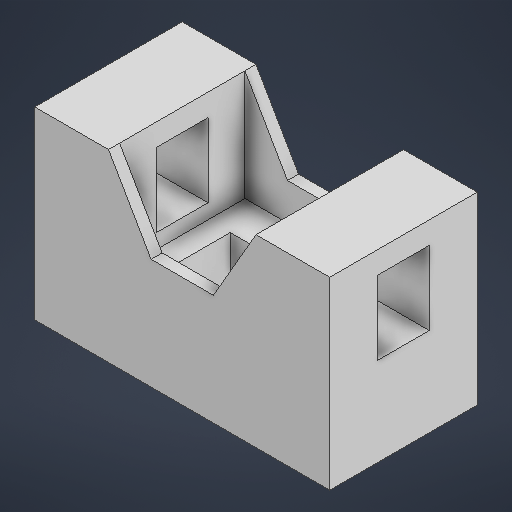
# Autodesk Inventor part: uhelnik_30x30_M6
Saved by Autodesk Inventor 2025.1 (Build 291241000, 241)
## iProperties
Created: 2024-12-28
Part Number: uhelnik_30x30_M6
Material: Všeobecné
Document SubType Name: Modeling
Designer: lukas
Density: 1 g/cm^3
Appearance: Výchozí
Author: lukas
## iProperties of the stored document uhelnik_30x30_3D tisk.ipt
Created: 2024-12-28
Part Number: uhelnik_30x30_3D tisk
Material: Všeobecné
Document SubType Name: Modeling
Designer: lukas
Density: 1 g/cm^3
Appearance: Výchozí
Author: lukas
Autodesk Inventor part; units mm, degrees
ref_plane "YZ Plane" through (0, 0, 0) normal (1, 0, 0) x (0, 1, 0)
ref_plane "XZ Plane" through (0, 0, 0) normal (0, 1, 0) x (-1, 0, 0)
ref_plane "XY Plane" through (0, 0, 0) normal (0, 0, 1) x (1, 0, 0)
sketch "Náčrt1" plane through (0, 0, 0) normal (0, 0, 1) x (1, 0, 0)
  line L0 (0, 17.5) -> (0, -17.5) projected
  line L1 (-28, 0) -> (28, 0) projected
  line L2 (-20, 12.5) -> (20, 12.5)
  line L3 (20, 12.5) -> (20, -12.5)
  line L4 (20, -12.5) -> (-20, -12.5)
  line L5 (-20, -12.5) -> (-20, 12.5)
  point P0 (0, 0)
  dimension "d0" = 40
  dimension "d1" = 25
  constraints: 8 end point, 2 parallel, 1 horizontal, 1 perpendicular, 2 other
  measures "d0" distance of L3.end L4.end
  measures "d1" distance of L2.end L3.end
extrude "Vysunutí1" add sketch "Náčrt1" along normal mid plane 20
sketch "Náčrt2" plane through (-20, 12.5, -10) normal (0, 1, 0) x (1, 0, 0)
  line L0 (0, 0) -> (40, 0) projected
  line L1 (0, 0) -> (0, -20) projected
  line L2 (40, -20) -> (0, -20) projected
  line L3 (40, 0) -> (40, -20) projected
  line L4 (-8, -10) -> (48, -10) projected
  line L5 (20, 4) -> (20, -24) projected
  line L6 (10, -18.5) -> (30, -18.5)
  line L7 (30, -18.5) -> (30, -1.5)
  line L8 (30, -1.5) -> (10, -1.5)
  line L9 (10, -1.5) -> (10, -18.5)
  point P0 (20, -10)
  dimension "d4" = 17
  dimension "d5" = 20
  constraints: 8 end point, 3 parallel, 1 horizontal, 1 perpendicular, 2 other
  measures "d4" distance of L8.end L6.start
  measures "d5" distance between parallel lines of L7 L9
extrude "Vysunutí2" cut sketch "Náčrt2" against normal blind 15 contours L8 L7 L4 L5 | L5 L4 L9 L8 | L4 L5 L6 L9 | L4 L7 L6 L5
sketch "Náčrt3" plane through (0, 0, 10) normal (0, 0, 1) x (1, 0, 0)
  line L0 (-20, -12.5) -> (20, -12.5) projected
  line L1 (20, -12.5) -> (20, 12.5) projected
  line L2 (20, 12.5) -> (-20, 12.5) projected
  line L3 (-20, 12.5) -> (-20, -12.5) projected
  line L4 (-10, 12.5) -> (-10, -2.5) projected
  line L5 (10, 12.5) -> (10, -2.5) projected
  line L6 (10, -2.5) -> (-10, -2.5) projected
  line L7 (-28, 0) -> (28, 0) projected
  line L8 (0, -17.5) -> (0, 17.5) projected
  line L9 (-10, 12.5) -> (-4.2265, 2.5)
  line L10 (-4.2265, 2.5) -> (4.2265, 2.5)
  line L11 (-20, 12.5) -> (20, 12.5) projected
  line L12 (4.2265, 2.5) -> (10, 12.5)
  line L13 (-10, 12.5) -> (10, 12.5)
  point P0 (0, 0)
  point P1 (0, 3.8397)
  dimension "d8" = 5
  dimension "d9" = 30
  dimension "d10" = 30
  constraints: 8 end point, 1 collinear, 1 parallel
  measures "d8" distance between parallel lines of L6 L10
  measures "d9" angle of L5 L12
  measures "d10" angle of L4 L9
extrude "Vysunutí3" cut sketch "Náčrt3" against normal through all contours L2 L8 L10 L9 | L8 L2 L12 L10
sketch "Náčrt5" plane through (20, -12.5, 10) normal (1, 0, 0) x (0, 0, -1)
  line L0 (20, 25) -> (0, 25) projected
  line L1 (0, 0) -> (0, 25) projected
  line L2 (20, 0) -> (0, 0) projected
  line L3 (20, 25) -> (20, 0) projected
  line L4 (18.5, 25) -> (18.5, 10) projected
  line L5 (18.5, 10) -> (1.5, 10) projected
  line L6 (1.5, 25) -> (1.5, 10) projected
  line L7 (10, -5) -> (10, 30) projected
  line L8 (-4, 12.5) -> (24, 12.5) projected
  line L9 (6.5, 22) -> (13.5, 22)
  line L10 (13.5, 22) -> (13.5, 12)
  line L11 (13.5, 12) -> (6.5, 12)
  line L12 (6.5, 12) -> (6.5, 22)
  line L13 (10, 22) -> (10, 12.5)
  line L14 (13.5, 12.5) -> (10, 12.5)
  line L15 (10, 22) -> (13.5, 22)
  line L16 (13.5, 12.5) -> (13.5, 22)
  dimension "d16" = 7
  dimension "d17" = 10
  dimension "d18" = 3
  constraints: 16 end point, 3 collinear, 2 horizontal, 2 parallel, 2 point on line, 1 midpoint, 1 perpendicular, 1 other
  measures "d16" distance of L10.end L11.end
  measures "d17" distance of L9.end L10.end
  measures "d18" distance between parallel lines of L0 L9
extrude "Vysunutí4" cut sketch "Náčrt5" against normal through all contours L9 L10 L8 L7 | L7 L8 L12 L9 | L10 L11 L7 L8 | L7 L11 L12 L8
sketch "Náčrt6" plane through (-20, -2.5, -10) normal (0, 1, 0) x (1, 0, 0)
  line L0 (30, -18.5) -> (10, -18.5) projected
  line L1 (30, -1.5) -> (30, -18.5) projected
  line L2 (10, -1.5) -> (30, -1.5) projected
  line L3 (10, -18.5) -> (10, -1.5) projected
  line L4 (-8, -10) -> (48, -10) projected
  line L5 (20, 4) -> (20, -24) projected
  line L6 (13, -6.5) -> (27, -6.5)
  line L7 (27, -6.5) -> (27, -13.5)
  line L8 (27, -13.5) -> (13, -13.5)
  line L9 (13, -13.5) -> (13, -6.5)
  point P0 (20, -10)
  dimension "d21" = 7
  dimension "d22" = 14
  dimension "d23" = 3
  constraints: 8 end point, 2 parallel, 1 horizontal, 1 perpendicular, 1 other
  measures "d21" distance of L6.end L7.end
  measures "d22" distance of L6.start L6.end
  measures "d23" distance between parallel lines of L3 L9
extrude "Vysunutí5" cut sketch "Náčrt6" against normal through all contours L8 L9 L4 L5 | L5 L4 L7 L8 | L4 L5 L6 L7 | L4 L9 L6 L5
